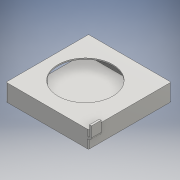
# Autodesk Inventor part: fan_sunon_ub3h3_500
Saved by Autodesk Inventor 2016 (Build 200138000, 138)
## iProperties
Created: 2016-08-08
Part Number: fan_sunon_ub3h3_500
Material: PC/ABS Plastic
Document SubType Name: Modeling
Designer: rawrdong
Density: 0.357273 g/cm^3
Appearance: Smooth - White
Author: rawrdong
Autodesk Inventor part; units mm, degrees
ref_plane "YZ Plane" through (0, 0, 0) normal (1, 0, 0) x (0, 1, 0)
ref_plane "XZ Plane" through (0, 0, 0) normal (0, 1, 0) x (-1, 0, 0)
ref_plane "XY Plane" through (0, 0, 0) normal (0, 0, 1) x (1, 0, 0)
sketch "master" plane through (0, 0, 0) normal (0, 0, 1) x (1, 0, 0)
  line L0 (-8.5, -8.5) -> (8.5, -8.5)
  line L1 (8.5, -8.5) -> (8.5, 8.5)
  line L2 (8.5, 8.5) -> (-8.5, 8.5)
  line L3 (-8.5, 8.5) -> (-8.5, -8.5)
  line L4 (-8.5, -8.5) -> (8.5, 8.5) construction
  line L5 (8.5, -8.5) -> (-8.5, 8.5) construction
  circle A0 centre (-0.65, 0) radius 5.65
  line L6 (5, 0) -> (8.5, 0) construction
  point P0 (0, 0)
  point P1 (0, 0)
  dimension "d1" = 11.3
  dimension "d0" = 17
  dimension "d12" = 3.5
  dimension "d14" = 9.15
  dimension "d22" = 0.65
  constraints: 14 end point, 4 midpoint, 2 horizontal, 2 horizontal alignment, 2 parallel, 2 perpendicular, 2 other
  measures "d0" distance of L0.end L1.end
  measures "d12" distance of L6.start L6.end
  measures "d14" distance from line of L1 point (-0.65, 0)
  measures "d22" distance of point (0, 0) point (-0.65, 0)
extrude "body" add sketch "master" against normal blind 3.5 contours L3 L2 L1 L0 | A0
sketch "Sketch2" plane through (-8.5, -8.5, 0) normal (-1, 0, 0) x (0, 0, 1)
  line L0 (0, 17) -> (0, 0) projected
  line L1 (0, 17) -> (-3.5, 17) projected
  line L2 (-3.5, 0) -> (-3.5, 17) projected
  line L3 (0, 0) -> (-3.5, 0) projected
  line L4 (0, 17) -> (0, 0) projected
  line L5 (-3, 16.16) -> (-0.25, 16.16)
  line L6 (-0.25, 16.16) -> (-0.25, 5.4)
  line L7 (-0.25, 5.4) -> (-3, 5.4)
  line L8 (-3, 5.4) -> (-3, 16.16)
  point P0 (0, 8.5)
  dimension "d4" = 5.4
  dimension "d5" = 0.84
  dimension "d6" = 0.25
  dimension "d7" = 0.5
  constraints: 8 end point, 2 parallel, 1 horizontal, 1 perpendicular
  measures "d4" distance between parallel lines of L3 L7
  measures "d5" distance between parallel lines of L1 L5
  measures "d6" distance between parallel lines of L0 L6
  measures "d7" distance between parallel lines of L2 L8
extrude "outlet" cut sketch "Sketch2" against normal blind 15 contours L5 L6 L7 L8
extrude "Extrusion3" cut sketch "master" against normal up to surface (3 mm away) contours A0
sketch "Sketch3" plane through (-8.5, -8.5, 0) normal (0, -1, 0) x (1, 0, 0)
  line L0 (17, 0) -> (17, -3.5) projected
  arc A0 (17, -1.75) -> (17.6, -1.15) centre (17, -1.15) ccw
  line L1 (17.6, -1.15) -> (17.6, 1)
  point P0 (8.5, 0)
  dimension "d15" = 1
  dimension "d16" = 0.6
  constraints: 2 end point, 2 point on circle, 1 centre point, 1 line through centre, 1 midpoint, 1 tangent, 1 vertical
  measures "d15" vertical distance of L0.start L1.end
  measures "d16" distance between parallel lines of L1 L0
sketch "Sketch4" plane through (8.5, -8.5, 0) normal (1, 0, 0) x (0, 0, -1)
  line L0 (1.35, 2) -> (1.35, 0)
  line L1 (1.35, 0) -> (1.75, 0)
  line L2 (1.75, 0) -> (1.75, 2)
  line L3 (1.75, 2) -> (1.35, 2)
  line L4 (1.35, 2) -> (1.75, 0) construction
  line L5 (1.35, 0) -> (1.75, 2) construction
  line L6 (0, 0) -> (3.5, 0) projected
  point P0 (0, 8.5)
  point P1 (1.55, 1)
  dimension "d17" = 2
  dimension "d18" = 0.4
  constraints: 12 end point, 3 midpoint, 2 parallel, 1 perpendicular, 1 vertical
  measures "d17" distance of L1.end L2.end
  measures "d18" distance of L2.end L0.start
sweep "Sweep1" add profiles "Sketch4" path "Sketch3" path curves A0 L1
fillet "Fillet1" radius 0.2 5 edges at (8.5, -8.5, -2.625) (8.5, 8.5, -1.75) (-8.5, -8.5, -1.75) (-8.5, 8.5, -1.75) (8.5, -8.5, -0.675)
body "Solid1"
